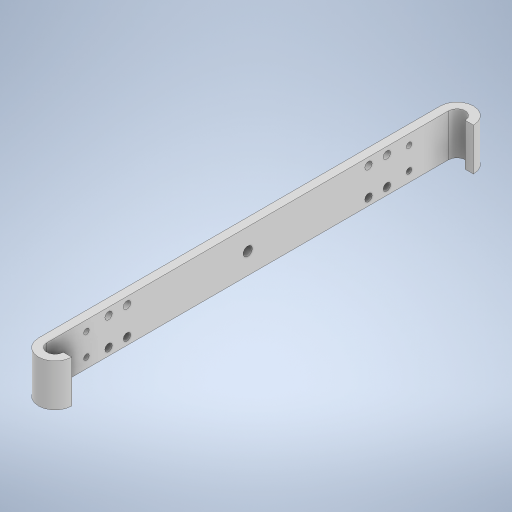
# Autodesk Inventor part: HUDSON-1-07 FRONT BUFFERR BEAM
Saved by Autodesk Inventor 2024.2 (Build 282272000, 272)
## iProperties
Created: 2024-10-05
Part Number: HUDSON-1-07 FRONT BUFFERR BEAM
Material: Generic
Document SubType Name: Modeling
Designer: Jimena Brenes
Density: 1 g/cm^3
Appearance: Default
Author: Jimena Brenes
Autodesk Inventor part; units mm, degrees
ref_plane "YZ Plane" through (0, 0, 0) normal (1, 0, 0) x (0, 1, 0)
ref_plane "XZ Plane" through (0, 0, 0) normal (0, 1, 0) x (-1, 0, 0)
ref_plane "XY Plane" through (0, 0, 0) normal (0, 0, 1) x (1, 0, 0)
sketch "Sketch1" plane through (0, 0, 0) normal (0, 1, 0) x (-1, 0, 0)
  line L0 (0, 0) -> (0, -218)
  arc A0 (0, 0) -> (-9, 0) centre (-4.5, 0) ccw
  line L1 (-9, 0) -> (-13.5, 0)
  line L2 (4.5, 0) -> (4.5, -218)
  arc A1 (4.5, 0) -> (-13.5, 0) centre (-4.5, 0) ccw
  line L3 (0, 0) -> (-17, 0) construction
  line L4 (52, -109) -> (-119, -109) construction
  line L5 (0, -218) -> (0, 0)
  arc A2 (-9, -218) -> (0, -218) centre (-4.5, -218) ccw
  line L6 (-9, -218) -> (-13.5, -218)
  line L7 (4.5, -218) -> (4.5, 0)
  arc A3 (-13.5, -218) -> (4.5, -218) centre (-4.5, -218) ccw
  point P0 (4.5, -109)
  dimension "d0" = 218
  dimension "d1" = 9
  dimension "d2" = 4.5
  dimension "d3" = 218
  dimension "d4" = 4.5
  dimension "d5" = 9
  dimension "d6" = 4.5
  dimension "d7" = 18
  constraints: 16 end point, 8 point on circle, 8 symmetric about line, 4 centre point, 2 horizontal, 2 point on line, 2 vertical, 1 midpoint, 1 parallel, 1 perpendicular, 1 tangent, 2 other
  measures "d0" distance of L0.start L0.end
  measures "d1" diameter of A0
  measures "d2" distance of L1.start L1.end
  measures "d3" distance of L2.start L2.end
  measures "d4" distance between parallel lines of L0 L2
  measures "d5" radius of A1
  measures "d6" radial gap between concentric circles of A0 A1
  measures "d7" distance of L1.end L2.start
extrude "Extrusion1" add sketch "Sketch1" along normal blind 23
sketch "Sketch2" plane through (0, 0, 0) normal (1, 0, 0) x (0, 0, -1)
  circle A0 centre (109, 11.5) radius 2.5
  line L0 (0, 23) -> (218, 23) projected
  line L1 (0, 0) -> (0, 23) projected
  line L2 (33.5, 4) -> (43.5, 4) construction
  line L3 (43.5, 4) -> (43.5, 19) construction
  line L4 (43.5, 19) -> (33.5, 19) construction
  line L5 (33.5, 19) -> (33.5, 4) construction
  line L6 (33.5, 4) -> (43.5, 19) construction
  line L7 (43.5, 4) -> (33.5, 19) construction
  circle A1 centre (43.5, 19) radius 2
  circle A2 centre (33.5, 19) radius 2
  circle A3 centre (33.5, 4) radius 2
  circle A4 centre (43.5, 4) radius 2
  line L8 (0, 0) -> (218, 0) projected
  line L9 (21.5, 5.5) -> (21.5, 17.5) construction
  circle A5 centre (21.5, 17.5) radius 1.5
  circle A6 centre (21.5, 5.5) radius 1.5
  line L10 (109, 37.5143) -> (109, -14.5143) construction
  line L11 (184.5, 4) -> (174.5, 4) construction
  line L12 (174.5, 4) -> (174.5, 19) construction
  line L13 (174.5, 19) -> (184.5, 19) construction
  line L14 (184.5, 19) -> (184.5, 4) construction
  line L15 (184.5, 4) -> (174.5, 19) construction
  line L16 (174.5, 4) -> (184.5, 19) construction
  circle A7 centre (174.5, 19) radius 2
  circle A8 centre (184.5, 19) radius 2
  circle A9 centre (184.5, 4) radius 2
  circle A10 centre (174.5, 4) radius 2
  line L17 (196.5, 5.5) -> (196.5, 17.5) construction
  circle A11 centre (196.5, 17.5) radius 1.5
  circle A12 centre (196.5, 5.5) radius 1.5
  point P0 (38.5, 11.5)
  point P1 (179.5, 11.5)
  dimension "d10" = 5
  dimension "d11" = 11.5
  dimension "d12" = 109
  dimension "d13" = 4
  dimension "d14" = 4
  dimension "d15" = 4
  dimension "d16" = 4
  dimension "d17" = 4
  dimension "d18" = 4
  dimension "d19" = 65.5
  dimension "d20" = 10
  dimension "d21" = 3
  dimension "d22" = 3
  dimension "d23" = 5.5
  dimension "d24" = 5.5
  dimension "d25" = 12
  constraints: 30 end point, 13 centre point, 13 coincident, 13 symmetric about line, 3 midpoint, 2 parallel, 2 vertical, 1 horizontal, 1 perpendicular, 6 other
  measures "d10" diameter of A0
  measures "d11" distance from line of L0 A0.centre
  measures "d12" distance from line of L1 A0.centre
  measures "d13" diameter of A1
  measures "d14" diameter of A2
  measures "d15" diameter of A3
  measures "d16" diameter of A4
  measures "d17" distance from line of L8 L2.end
  measures "d18" distance from line of L0 L3.end
  measures "d19" horizontal distance of L2.end A0.centre
  measures "d20" distance of L2.end L2.start
  measures "d21" diameter of A5
  measures "d22" diameter of A6
  measures "d23" distance from line of L0 L9.end
  measures "d24" distance from line of L8 L9.start
  measures "d25" horizontal distance of A3.centre A6.centre
hole "Hole1" at (0, 17.5, -21.5) at (0, 5.5, -21.5) at (0, 17.5, -196.5) at (0, 5.5, -196.5) direction (-1, 0, 0) diameter 3 end through all
hole "Hole2" at (0, 19, -184.5) at (0, 19, -174.5) at (0, 4, -184.5) at (0, 4, -174.5) at (0, 19, -33.5) at (0, 19, -43.5) at (0, 4, -33.5) at (0, 4, -43.5) direction (-1, 0, 0) diameter 4 end through all
hole "Hole3" at (0, 11.5, -109) direction (-1, 0, 0) diameter 5 end through all
body "Solid1"
